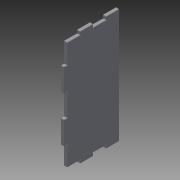
# Autodesk Inventor part: cajon front grande
Saved by Autodesk Inventor 2015 (Build 190159000, 159)
## iProperties
Created: 2016-01-27
Part Number: cajon front grande
Material: Generic
Document SubType Name: Modeling
Designer: iberopuebla
Density: 1 g/cm^3
Appearance: Default
Author: iberopuebla
Autodesk Inventor part; units mm, degrees
ref_plane "YZ Plane" through (0, 0, 0) normal (1, 0, 0) x (0, 1, 0)
ref_plane "XZ Plane" through (0, 0, 0) normal (0, 1, 0) x (-1, 0, 0)
ref_plane "XY Plane" through (0, 0, 0) normal (0, 0, 1) x (1, 0, 0)
sketch "Sketch1" plane through (0, 0, 0) normal (1, 0, 0) x (0, 1, 0)
  line L0 (75, 0) -> (150, 0)
  line L1 (-2.4984, -131.9115) -> (-17.9998, -131.9115)
  line L2 (-2.4984, -263.9115) -> (-17.9998, -263.9115)
  line L3 (-17.9998, -131.9115) -> (-17.9998, -263.9115)
  line L4 (0, -129.5) -> (0, -18)
  line L5 (75, -15.5) -> (75, 0)
  line L6 (152.5, -18) -> (222.5, -18)
  line L7 (225, 0) -> (300, 0)
  arc A0 (222.5, -18) -> (225, -15.5) centre (225, -18) ccw
  arc A1 (150, -15.5) -> (152.5, -18) centre (150, -18) ccw
  arc A2 (72.5, -18) -> (75, -15.5) centre (75, -18) ccw
  line L8 (150, 0) -> (150, -15.5)
  line L9 (72.5, -18) -> (0, -18)
  line L10 (225, 0) -> (225, -15.5)
  arc A3 (-2.4984, -131.9115) -> (0, -129.5) centre (0, -132) ccw
  arc A4 (0.0002, -266.5) -> (-2.4984, -263.9115) centre (0, -264) ccw
  arc A5 (0, -530.5) -> (-2.4984, -528.0885) centre (0, -528) ccw
  line L11 (0, -530.5) -> (0, -642)
  line L12 (75, -660) -> (150, -660)
  arc A6 (-2.4984, -396.0885) -> (0.0002, -393.5) centre (0, -396) ccw
  line L13 (-17.9998, -528.0885) -> (-17.9998, -396.0885)
  line L14 (-2.4984, -528.0885) -> (-17.9998, -528.0885)
  arc A7 (75, -644.5) -> (72.5, -642) centre (75, -642) ccw
  line L15 (75, -644.5) -> (75, -660)
  arc A8 (152.5, -642) -> (150, -644.5) centre (150, -642) ccw
  line L16 (150, -660) -> (150, -644.5)
  line L17 (152.5, -642) -> (222.5, -642)
  arc A9 (225, -644.5) -> (222.5, -642) centre (225, -642) ccw
  line L18 (225, -660) -> (225, -644.5)
  line L19 (225, -660) -> (300, -660)
  line L20 (-2.4984, -396.0885) -> (-17.9998, -396.0885)
  line L21 (72.5, -642) -> (0, -642)
  line L22 (300, 0) -> (300, -660)
  line L23 (0.0002, -266.5) -> (0.0002, -393.5)
  point P0 (0, 0)
  point P1 (0, 0)
  point P2 (0, -660)
  dimension "d0" = 132
  dimension "d1" = 5
  dimension "d2" = 5
  dimension "d3" = 5
  dimension "d4" = 18
  dimension "d5" = 18
  dimension "d6" = 18
  dimension "d7" = 18
  dimension "d8" = 18
  dimension "d9" = 5
  dimension "d10" = 5
  dimension "d11" = 18
  dimension "d12" = 18
  dimension "d13" = 132
  dimension "d14" = 75
  dimension "d15" = 75
  dimension "d16" = 75
  dimension "d17" = 18
  dimension "d18" = 18
  dimension "d19" = 18
  dimension "d20" = 17.9998
  dimension "d21" = 660
  constraints: 48 end point, 20 point on circle, 11 vertical, 10 centre point, 8 horizontal, 3 perpendicular, 2 vertical alignment, 1 parallel, 29 other
  measures "d0" distance between parallel lines of L2 L1
  measures "d1" diameter of A0
  measures "d2" diameter of A1
  measures "d3" diameter of A2
  measures "d4" distance of L7.start A0.centre
  measures "d5" distance of A1.centre L0.end
  measures "d6" distance of L0.start A2.centre
  measures "d7" vertical distance of L9.start L0.start
  measures "d8" distance between parallel lines of L7 L6
  measures "d9" diameter of A3
  measures "d10" diameter of A4
  measures "d11" distance of L2.end A4.centre
  measures "d12" distance of A3.centre L1.end
  measures "d13" distance of A3.centre A4.centre
  measures "d14" distance between parallel lines of L8 L10
  measures "d15" distance between parallel lines of L5 L8
  measures "d16" distance from line of point (0, 0) L5
  measures "d17" distance from line of L9 point (0, 0)
  measures "d18" vertical distance of point (0, 0) A2.centre
  measures "d19" distance between parallel lines of L6 L0
  measures "d20" distance between parallel lines of L4 L3
  measures "d21" distance of L7.end L19.end
extrude "Extrusion1" add sketch "Sketch1" along normal blind 18
body "Solid1"
